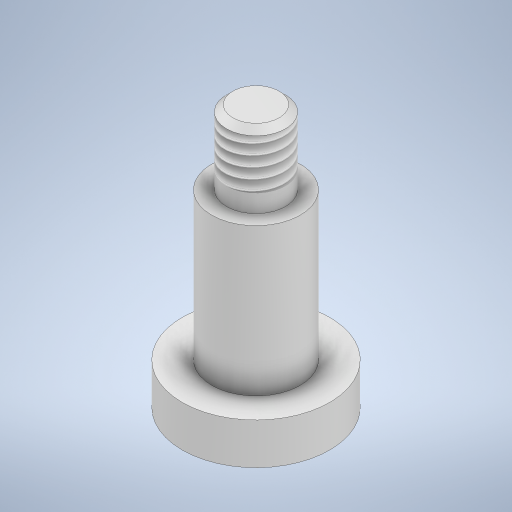
# Autodesk Inventor part: DBTSY4-10-5-DHC
Saved by Autodesk Inventor 2024.2 (Build 282272000, 272)
## iProperties
Created: 2024-01-06
Part Number: DBTSY4-10-5-DHC
Material: Stainless Steel AISI 304
Document SubType Name: Modeling
Designer: Masato Kubotera
Density: 8 g/cm^3
Appearance: Satin
Mass: 4.42866 g
Surface Area: 5.10286 cm^2
Volume: 0.553583 cm^3
Catalog Web Link: https://jp.misumi-ec.com/vona2/detail/110302403310/?ProductCode=DBSY4-10-5
Vendor: MISUMI
Author: Masato Kubotera
Autodesk Inventor part; units mm, degrees
ref_plane "YZ Plane" through (0, 0, 0) normal (1, 0, 0) x (0, 1, 0)
ref_plane "XZ Plane" through (0, 0, 0) normal (0, 1, 0) x (-1, 0, 0)
ref_plane "XY Plane" through (0, 0, 0) normal (0, 0, 1) x (1, 0, 0)
sketch "Sketch1" plane through (0, 0, 0) normal (0, 1, 0) x (-1, 0, 0)
  line L0 (0, 0) -> (0, 17.8)
  line L1 (0, 17.8) -> (-2, 17.8)
  line L2 (-2, 17.8) -> (-2, 12.8)
  line L3 (-2, 12.8) -> (-3, 12.8)
  line L4 (-3, 12.8) -> (-3, 2.8)
  line L5 (-3, 2.8) -> (-5, 2.8)
  line L6 (-5, 2.8) -> (-5, 0)
  line L7 (-5, 0) -> (0, 0)
  dimension "d0" = 10
  dimension "d1" = 6
  dimension "d2" = 4
  dimension "d3" = 5
  dimension "d4" = 10
  dimension "d5" = 2.8
  constraints: 16 end point, 4 horizontal, 4 vertical
  measures "d0" diameter of L6 L0
  measures "d1" diameter of L4 L0
  measures "d2" diameter of L2 L0
  measures "d3" distance of L1.end L2.end
  measures "d4" distance of L3.end L4.end
  measures "d5" distance of L5.end L6.end
revolve "Revolution1" add sketch "Sketch1" angle 360 about axis through (0, 0, 0) along (0, 0, 1)
thread "Thread1" size "M4x0.7" class "6g" standard "ANSI Metric M Profile" length 6 offset 1.2
sketch "Sketch2" plane through (0, 0, 0) normal (0, 0, -1) x (-1, 0, 0)
  line L0 (0, 1.4434) -> (1.25, 0.7217)
  line L1 (1.25, 0.7217) -> (1.25, -0.7217)
  line L2 (1.25, -0.7217) -> (0, -1.4434)
  line L3 (0, -1.4434) -> (-1.25, -0.7217)
  line L4 (-1.25, -0.7217) -> (-1.25, 0.7217)
  line L5 (-1.25, 0.7217) -> (0, 1.4434)
  point P0 (0, 0)
  point P1 (0, 0)
  dimension "d9" = 2.5
  constraints: 12 end point, 1 coincident, 1 vertical, 13 other
  measures "d9" distance between parallel lines of L1 L4
extrude "Extrusion1" cut sketch "Sketch2" against normal blind 2
chamfer "Chamfer1" distance 0.43 angle 45 1 edges at (-2, 0, 17.8)
body "Solid1"
